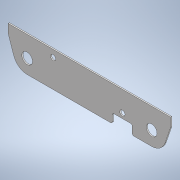
# Autodesk Inventor part: outside_plate
Saved by Autodesk Inventor 2022 (Build 260153000, 153)
## iProperties
Created: 2021-07-14
Part Number: outside_plate
Material: Generic
Document SubType Name: Modeling
Designer: gfellows
Density: 1 g/cm^3
Appearance: Default
Author: gfellows
Autodesk Inventor part; units mm, degrees
ref_plane "YZ Plane" through (0, 0, 0) normal (1, 0, 0) x (0, 1, 0)
ref_plane "XZ Plane" through (0, 0, 0) normal (0, 1, 0) x (-1, 0, 0)
ref_plane "XY Plane" through (0, 0, 0) normal (0, 0, 1) x (1, 0, 0)
sketch "main_sketch" plane through (0, 0, 0) normal (0, 0, 1) x (1, 0, 0)
  circle A0 centre (0, 0) radius 50 construction
  circle A1 centre (330.2, 0) radius 50 construction
  circle A2 centre (0, 0) radius 12.7 construction
  circle A3 centre (330.2, 0) radius 12.7 construction
  circle A4 centre (68.8579, 36.0008) radius 12.7 construction
  circle A5 centre (252.6541, 0.2) radius 12.7 construction
  line L0 (68.8579, 36.0008) -> (0, 0) construction
  circle A6 centre (68.8579, 36.0008) radius 6.75 construction
  circle A7 centre (252.6541, 0.2) radius 6.75 construction
  line L1 (96.8579, 55) -> (220.7349, 55) construction
  line L2 (220.7349, 55) -> (220.7349, 17.0016) construction
  line L3 (220.7349, 17.0016) -> (96.8579, 17.0016) construction
  line L4 (96.8579, 17.0016) -> (96.8579, 55) construction
  line L5 (224.6541, -18.7992) -> (100.7771, -18.7992) construction
  line L6 (100.7771, -18.7992) -> (100.7771, 19.1992) construction
  line L7 (100.7771, 19.1992) -> (224.6541, 19.1992) construction
  line L8 (224.6541, 19.1992) -> (224.6541, -18.7992) construction
  line L9 (100.7771, 0.2) -> (224.6541, 0.2) construction
  line L10 (96.8579, 36.0008) -> (220.7349, 36.0008) construction
  line L11 (330.1672, -12.7) -> (252.6213, -12.5) construction
  line L12 (5.8842, -11.2546) -> (74.7421, 24.7462) construction
  line L13 (-5.8842, 11.2546) -> (62.9737, 47.2554) construction
  line L14 (253.6541, -13.3) -> (277.6541, -13.3) construction
  line L15 (277.6541, -13.3) -> (277.6541, -37.3) construction
  line L16 (277.6541, -37.3) -> (253.6541, -37.3) construction
  line L17 (253.6541, -37.3) -> (253.6541, -13.3) construction
  line L18 (252.6541, 0.2) -> (330.2, 0) construction
  line L19 (0, -50) -> (330.2, -50) construction
  line L20 (250.6541, -37.3) -> (226.6541, -37.3) construction
  line L21 (226.6541, -37.3) -> (226.6541, -13.3) construction
  line L22 (226.6541, -13.3) -> (250.6541, -13.3) construction
  line L23 (250.6541, -13.3) -> (250.6541, -37.3) construction
  line L24 (-50, 58.175) -> (380.2, 58.175) construction
  line L25 (380.2, 58.175) -> (380.2, 55) construction
  line L26 (380.2, 55) -> (-50, 55) construction
  line L27 (-50, 55) -> (-50, 58.175) construction
  line L28 (252.6868, 12.9) -> (330.2328, 12.7) construction
  line L29 (224.6541, 9.7) -> (238.5511, 9.7) construction
  line L30 (238.5511, 9.7) -> (238.5511, -9.3) construction
  line L31 (238.5511, -9.3) -> (224.6541, -9.3) construction
  line L32 (224.6541, -9.3) -> (224.6541, 9.7) construction
  line L33 (225.6541, -12.3) -> (278.6541, -12.3)
  line L34 (278.6541, -12.3) -> (278.6541, -37.3)
  line L35 (225.6541, -12.3) -> (225.6541, -37.3)
  line L36 (317.9464, 55) -> (342.9, 55) construction
  line L37 (342.9, 55) -> (342.9, 50) construction
  line L38 (342.9, 50) -> (317.9464, 50) construction
  line L39 (317.9464, 50) -> (317.9464, 55) construction
  line L40 (380.2, 55) -> (380.2, -5.9093) construction
  line L41 (-50, 55) -> (-50, 17.1992) construction
  line L42 (-50, 55) -> (380.2, 55) construction
  line L43 (-50, 55) -> (380.2, 55)
  circle A8 centre (330.2, 0) radius 14.2748
  circle A9 centre (0, 0) radius 14.2748
  circle A10 centre (252.6541, 0.2) radius 7.008
  circle A11 centre (68.8579, 36.0008) radius 7.008
  circle A12 centre (330.2, 0) radius 37.3
  circle A13 centre (0, 0) radius 37.3
  line L44 (380.2, 52.5) -> (380.2, 43) projected
  line L45 (380.2, 55) -> (380.2, 31)
  line L46 (380.2, 31) -> (365.4988, -12.0533)
  line L47 (278.6541, -37.3) -> (330.2, -37.3)
  line L48 (-50, 55) -> (-50, 31)
  line L49 (-50, 31) -> (-35.2988, -12.0533)
  line L50 (225.6541, -37.3) -> (0, -37.3)
  circle A14 centre (296.2, 47) radius 2 projected
  circle A15 centre (304.2, 47) radius 2 projected
  circle A16 centre (312.2, 47) radius 2 projected
  circle A17 centre (320.2, 47) radius 2 projected
  circle A18 centre (328.2, 47) radius 2 projected
  circle A19 centre (336.2, 47) radius 2 projected
  circle A20 centre (344.2, 47) radius 2 projected
  circle A21 centre (352.2, 47) radius 2 projected
  circle A22 centre (360.2, 47) radius 2 projected
  circle A23 centre (368.2, 47) radius 2 projected
  circle A24 centre (376.2, 47) radius 2 projected
  circle A25 centre (-46, 47) radius 2 projected
  circle A26 centre (-38, 47) radius 2 projected
  circle A27 centre (-30, 47) radius 2 projected
  circle A28 centre (-22, 47) radius 2 projected
  circle A29 centre (-6, 47) radius 2 projected
  circle A30 centre (-14, 47) radius 2 projected
  circle A31 centre (2, 47) radius 2 projected
  circle A32 centre (10, 47) radius 2 projected
  circle A33 centre (18, 47) radius 2 projected
  circle A34 centre (26, 47) radius 2 projected
  circle A35 centre (34, 47) radius 2 projected
  circle A36 centre (283.6541, -32.3) radius 4
  circle A37 centre (283.6541, -32.3) radius 2
  line L51 (272.6868, 22.9) -> (272.6868, 2.9) construction
  line L52 (270.6868, 22.9) -> (270.6868, 2.9)
  line L53 (274.6868, 2.9) -> (274.6868, 22.9)
  arc A38 (274.6868, 22.9) -> (270.6868, 22.9) centre (272.6868, 22.9) ccw
  arc A39 (270.6868, 2.9) -> (274.6868, 2.9) centre (272.6868, 2.9) ccw
  line L54 (61.6516, 6.6178) -> (52.3851, 24.3416) construction
  line L55 (63.4239, 7.5445) -> (54.1575, 25.2683)
  line L56 (50.6127, 23.415) -> (59.8792, 5.6912)
  arc A40 (59.8792, 5.6912) -> (63.4239, 7.5445) centre (61.6516, 6.6178) ccw
  arc A41 (54.1575, 25.2683) -> (50.6127, 23.415) centre (52.3851, 24.3416) ccw
  circle A42 centre (209.6541, -28.0496) radius 4
  line L57 (221.9902, -18.7992) -> (221.9902, -37.3)
  circle A43 centre (161.6541, -28.0496) radius 4
  circle A44 centre (113.6541, -28.0496) radius 4
  circle A45 centre (65.6541, -28.0496) radius 4
  circle A46 centre (209.6541, -28.0496) radius 2
  circle A47 centre (161.6541, -28.0496) radius 2
  circle A48 centre (113.6541, -28.0496) radius 2
  circle A49 centre (65.6541, -28.0496) radius 2
  circle A50 centre (252.6541, 36.0008) radius 4
  circle A51 centre (252.6541, 36.0008) radius 2
  point P0 (238.5511, 0.2)
  point P1 (272.6868, 12.9)
  point P2 (57.0183, 15.4797)
  point P3 (221.9902, -28.0496)
  dimension "d0" = 100
  dimension "d1" = 100
  dimension "d2" = 25.4
  dimension "d3" = 25.4
  dimension "d4" = 25.4
  dimension "d5" = 25.4
  dimension "d6" = 13.5
  dimension "d7" = 13.5
  dimension "d8" = 37.9984
  dimension "d9" = 37.9984
  dimension "d10" = 24
  dimension "d11" = 24
  dimension "d12" = 77.5462
  dimension "d13" = 330.2
  dimension "d14" = 123.877
  dimension "d15" = 123.877
  dimension "d16" = 28
  dimension "d17" = 28
  dimension "d18" = 77.7011
  dimension "d19" = 12.7
  dimension "d20" = 24
  dimension "d21" = 3.175
  dimension "d23" = 12.7
  dimension "d24" = 3
  dimension "d25" = 19
  dimension "d26" = 1
  dimension "d27" = 1
  dimension "d28" = 1
  dimension "d29" = 1
  dimension "d32" = 5
  dimension "d34" = 3
  dimension "d40" = 28.5496
  dimension "d41" = 28.5496
  dimension "d42" = 14.016
  dimension "d43" = 14.016
  dimension "d45" = 24
  dimension "d46" = 24
  dimension "d48" = 8
  dimension "d49" = 5
  dimension "d50" = 5
  dimension "d51" = 4
  dimension "d52" = 4
  dimension "d53" = 20
  dimension "d54" = 20
  dimension "d55" = 4
  dimension "d56" = 20
  dimension "d57" = 18
  dimension "d58" = 8
  dimension "d59" = 16
  dimension "d62" = 48
  dimension "d67" = 4
  dimension "d68" = 4
  dimension "d69" = 4
  dimension "d70" = 4
  dimension "d71" = 8
  dimension "d72" = 4
  constraints: 118 end point, 28 centre point, 20 point on circle, 20 tangent, 17 coincident, 17 equal length, 13 horizontal, 10 horizontal alignment, 9 perpendicular, 9 vertical, 8 midpoint, 6 point on line, 4 vertical alignment, 10 other
  measures "d2" diameter of A2
  measures "d3" diameter of A3
  measures "d4" diameter of A4
  measures "d5" diameter of A5
  measures "d6" diameter of A6
  measures "d7" diameter of A7
  measures "d8" distance between parallel lines of L1 L3
  measures "d9" distance between parallel lines of L5 L7
  measures "d10" distance of L15.end L16.end
  measures "d11" distance of L14.end L15.end
  measures "d12" distance of point (330.2, 0) A5.centre
  measures "d13" distance of point (330.2, 0) point (0, 0)
  measures "d14" distance of L5.start L5.end
  measures "d15" distance of L1.start L1.end
  measures "d16" distance from line of L8 A5.centre
  measures "d17" distance from line of L4 L0.start
  measures "d18" distance of L0.start L0.end
  measures "d19" distance between parallel lines of L19 L16
  measures "d20" distance of L20.start L20.end
  measures "d21" distance of L25.end L24.end
  measures "d23" distance between parallel lines of L19 L20
  measures "d24" distance between parallel lines of L17 L23
  measures "d25" distance of L29.end L30.end
  measures "d26" distance between parallel lines of L21 L35
  measures "d27" distance between parallel lines of L35 L8
  measures "d28" distance between parallel lines of L33 L22
  measures "d29" horizontal distance of L14.end L33.end
  measures "d32" distance of L36.end L37.end
  measures "d34" distance between parallel lines of L33 L31
  measures "d40" diameter of A8
  measures "d41" diameter of A9
  measures "d42" diameter of A10
  measures "d43" diameter of A11
  measures "d45" distance of L25.end L45.end
  measures "d46" distance of L26.end L48.end
  measures "d48" diameter of A36
  measures "d49" distance from line of L47 A36.centre
  measures "d50" distance from line of L34 A36.centre
  measures "d51" diameter of A37
  measures "d52" diameter of A39
  measures "d53" distance of L52.start L52.end
  measures "d54" distance of L28.start point (272.687, 12.9)
  measures "d55" diameter of A41
  measures "d56" distance of L56.start L56.end
  measures "d57" distance from line of L12.end L55
  measures "d58" diameter of A42
  measures "d59" distance from line of L35 A42.centre
  measures "d62" distance of A42.centre A43.centre
  measures "d67" diameter of A46
  measures "d68" diameter of A47
  measures "d69" diameter of A48
  measures "d70" diameter of A49
  measures "d71" diameter of A50
  measures "d72" diameter of A51
extrude "Extrusion1" add sketch "main_sketch" along normal blind 3.175 contours L35 L50 A13 L49 L48 L43 L45 L44 L46 A12 L47 L34 L33 | A12 | A13 | A36 | A42 | A43 | A44 | A45 | A50
fillet "Fillet4" radius 4 4 edges at (278.6541, -37.3, 1.5875) (278.6541, -12.3, 1.5875) (225.6541, -12.3, 1.5875) (225.6541, -37.3, 1.5875)
fillet "Fillet5" radius 8 2 edges at (-50, 31, 1.5875) (380.2, 31, 1.5875)
equation "\"d9\" = d8"
equation "\"d15\" = d14"
equation "\"d20\" = d10"
body "Solid1"
